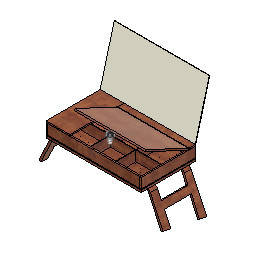
capstone new final (Autodesk Fusion 360 design; units mm, degrees)
Autodesk Fusion 360 part; units mm, degrees
note: some values were not read from the file. Set by a fixed rule: which face or edge a step refers to.
sketch "Sketch1" plane through (0, 0, 0) normal (0, 1, 0) x (1, 0, 0)
  line L0 (0, 0) -> (177.8, 0)
  line L1 (177.8, 0) -> (177.8, -406.4)
  line L2 (177.8, -406.4) -> (0, -406.4)
  line L3 (0, -406.4) -> (0, 0)
  dimension "d1" = 177.8
  dimension "d2" = 406.4
  constraint horizontal L0
  constraint vertical L1
  constraint horizontal L2
  constraint vertical L3
  constraint coincident L0.start L3.end
  measures "d1" distance of L0.start L0.end
  measures "d2" distance of L0.start L2.end
extrude "Extrude1" add sketch "Sketch1" along normal blind 12 makes body 1
extrude "Extrude2" add 1 faces at (177.8, 4, 135.4667) along direction (1, 0, 0) blind 533.4 separate body on bodies 1 makes body 2
move_face "OffsetFaces1" offset -50.8 1 faces at (355.6, 4, 0) on bodies 2
extrude "Extrude3" add 1 faces at (355.6, 4, 50.8) along direction (0, 0, -1) blind 50.8 separate body on bodies 2 makes body 3
sketch "Sketch2" plane through (0, 0, 0) normal (0, -1, 0) x (1, 0, 0)
  line L0 (177.8, 406.4) -> (0, 406.4)
  line L1 (0, 406.4) -> (0, 0)
  line L2 (0, 0) -> (177.8, 0)
  line L3 (177.8, 0) -> (177.8, 406.4)
  line L4 (0, 406.4) -> (12, 406.4)
  line L5 (12, 406.4) -> (12, 0)
  line L6 (12, 0) -> (0, 0)
  line L7 (0, 0) -> (0, 406.4)
  dimension "d10" = 12
  dimension "d11" = 406.4
  constraint horizontal L4
  constraint vertical L5
  constraint horizontal L6
  constraint vertical L7
  constraint coincident L0.end L1.start
  measures "d10" distance of L0.end L4.end
  measures "d11" distance of L0.end L1.end
extrude "Extrude4" add sketch "Sketch2" along normal blind 76.2 separate body contours L0 L1 L2 L4 L5 L6 L7 makes body 4
ref_plane "WorkPlane1" through (355.6, 6, 203.2) normal (-1, 0, 0) x (0, 0, 1)
mirror "Mirror1" about plane through (355.6, 6, 203.2) normal (-1, 0, 0) of bodies 4 makes body 5
sketch "Sketch3" plane through (0, 0, 0) normal (0, -1, 0) x (1, 0, 0)
  line L0 (711.2, 50.8) -> (177.8, 50.8)
  line L1 (177.8, 50.8) -> (177.8, 0)
  line L2 (177.8, 0) -> (711.2, 0)
  line L3 (711.2, 0) -> (711.2, 50.8)
  line L4 (0, 0) -> (36.2396, 0)
  line L5 (36.2396, 0) -> (36.2396, 369.3683)
  line L6 (36.2396, 369.3683) -> (0, 369.3683)
  line L7 (0, 369.3683) -> (0, 0)
  line L8 (20.6379, 405.3508) -> (675.3287, 405.3508)
  line L9 (675.3287, 405.3508) -> (675.3287, 393.3508)
  line L10 (675.3287, 393.3508) -> (20.6379, 393.3508)
  line L11 (20.6379, 393.3508) -> (20.6379, 405.3508)
  line L12 (11.8338, 405.3508) -> (698.3946, 405.3508)
  line L13 (698.3946, 405.3508) -> (698.3946, 393.3508)
  line L14 (698.3946, 393.3508) -> (11.8338, 393.3508)
  line L15 (11.8338, 393.3508) -> (11.8338, 405.3508)
  dimension "d16" = 12
  constraint horizontal L4
  constraint vertical L5
  constraint horizontal L6
  constraint vertical L7
  constraint coincident L4.start L7.end
  constraint horizontal L8
  constraint vertical L9
  constraint horizontal L10
  constraint vertical L11
  constraint horizontal L12
  constraint vertical L13
  constraint horizontal L14
  constraint vertical L15
  measures "d16" distance of L8 L10
extrude "Extrude5" add sketch "Sketch3" along normal blind 76.2 separate body contours L8 L9 L10 L11 L12 L14 | L11 L12 L14 L15 | L9 L12 L13 L14 makes body 6
ref_plane "WorkPlane2" through (444.5, 6, 203.2) normal (0, 0, -1) x (-1, 0, 0)
mirror "Mirror2" about plane through (444.5, 6, 203.2) normal (0, 0, -1) of bodies 6 makes body 7
sketch "Sketch4" plane through (0, 0, 0) normal (0, 1, 0) x (1, 0, 0)
ref_plane "WorkPlane3" through (355.1142, -38.1, 7.0492) normal (0, 1, 0) x (-1, 0, 0)
sketch "Sketch5" plane through (0, 0, 0) normal (0, 1, 0) x (1, 0, 0)
  line L0 (472.5788, 451.5753) -> (-238.6212, 451.5753)
  line L1 (-238.6212, 451.5753) -> (-238.6212, 45.1753)
  line L2 (-238.6212, 45.1753) -> (472.5788, 45.1753)
  line L3 (472.5788, 45.1753) -> (472.5788, 451.5753)
  dimension "d21" = 711.2
  dimension "d22" = 406.4
  constraint horizontal L0
  constraint vertical L1
  constraint horizontal L2
  constraint vertical L3
  measures "d21" distance of L0.start L0.end
  measures "d22" distance of L0.start L2.end
extrude "Extrude6" add sketch "Sketch5" along normal blind 6 separate body makes body 8
move_body "Move1" bodies 8 to x (1, 0, 0) y (0, 1, 0) z (0, 0, 1) at (0, -77.1672, 454.3724)
move_body "Move2" bodies 8 to x (1, 0, 0) y (0, 1, 0) z (0, 0, 1) at (239.8938, -5.0258, -3.112)
extrude "Extrude7" add 1 faces at (475.4059, -82.193, 270.6185) along direction (0, -1, 0) blind 18 separate body on bodies 8 makes body 9
move_body "Move3" bodies 8 9 to x (1, 0, 0) y (0, 1, 0) z (0, 0, 1) at (-1.8025, 0, 0)
sketch "Sketch6" plane through (0, -100.193, 0) normal (0, -1, 0) x (1, 0, 0)
  line L0 (710.6701, -0.3149) -> (710.6701, 406.0851)
  line L1 (710.6701, 406.0851) -> (-0.5299, 406.0851)
  line L2 (-0.5299, 406.0851) -> (-0.5299, -0.3149)
  line L3 (-0.5299, -0.3149) -> (710.6701, -0.3149)
  line L4 (-98.6513, -2.8621) -> (-403.4513, -2.8621)
  line L5 (-403.4513, -2.8621) -> (-403.4513, 47.5823)
  line L6 (-4.9831, -2.8621) -> (-55.7831, -2.8621)
  line L7 (-149.6797, 302.2068) -> (-403.6797, 302.2068)
  line L8 (-403.6797, 302.2068) -> (-403.6797, 248.7195)
  line L9 (-403.6797, 248.7195) -> (-304.5716, 248.7195)
  line L10 (-148.6459, 248.7195) -> (-140.733, 248.7195)
  line L11 (-148.6457, 48.2483) -> (-107.1833, 48.1456)
  line L12 (-253.7726, 248.4073) -> (-250.8436, 47.939)
  line L13 (-304.5716, 248.7195) -> (-304.5716, 50.2895)
  line L14 (-253.7726, 44.9279) -> (-253.7726, 248.4073)
  line L15 (-148.6459, 248.7195) -> (-253.7726, 248.4073)
  line L16 (-148.6457, 48.2483) -> (-253.7726, 44.9279)
  line L17 (-304.5716, 50.2895) -> (-403.4513, 47.5823)
  line L18 (-403.6797, 302.2068) -> (-149.6797, 302.2068)
  line L19 (-149.6797, 302.2068) -> (-140.733, 248.7195)
  line L20 (-107.1833, 48.1456) -> (-98.6513, -2.8621)
  line L21 (-304.5716, 50.2895) -> (-308.3744, 53.8896)
  line L22 (-304.5716, 248.7195) -> (-308.8143, 244.4768)
  line L23 (-253.7726, 248.4073) -> (-241.4018, 236.1097)
  line L24 (-253.7726, 44.9279) -> (-236.2729, 63.5691)
  circle A0 centre (-251.645, 246.2923) radius 3
  circle A1 centre (-306.6929, 246.5981) radius 3
  circle A2 centre (-306.7502, 52.3519) radius 3
  circle A3 centre (-251.7193, 47.1151) radius 3
  dimension "d27" = 304.8
  dimension "d29" = 50.8
  dimension "d63" = 50.8
  dimension "d64" = 203.4794
  dimension "d65" = 254
  dimension "d177" = 45
  dimension "d178" = 45
  dimension "d179" = 45
  dimension "d180" = 45
  dimension "d181" = 6
  dimension "d182" = 6
  dimension "d183" = 6
  dimension "d184" = 6
  constraint horizontal L4
  constraint vertical L5
  constraint horizontal L6
  constraint coincident L4 L6.start
  constraint horizontal L7
  constraint vertical L8
  constraint horizontal L9
  constraint collinear L9 L10
  constraint vertical L13
  constraint vertical L14
  constraint perpendicular L8 L18
  constraint collinear L19 L20
  constraint coincident L23 A0.centre
  constraint coincident L12.start A0
  constraint midpoint L22 A1.centre
  constraint coincident L9.end A1
  constraint coincident L21 A2.centre
  constraint coincident L13.end A2
  constraint coincident L24 A3.centre
  constraint coincident L14.start A3
  measures "d27" distance of L4.start L4.end
  measures "d29" distance of L6.start L6.end
  measures "d63" distance of L12.start L9.end
  measures "d64" distance of L12.start L14.start
  measures "d65" distance of L7.end L7.start
  measures "d177" angle of L17 L21
  measures "d178" angle of L16 L24
  measures "d179" angle of L15 L23
  measures "d180" angle of L13 L22
  measures "d181" diameter of A0
  measures "d182" diameter of A3
  measures "d183" diameter of A2
  measures "d184" diameter of A1
extrude "Extrude8" add sketch "Sketch6" along normal blind 18 separate body contours L4 L5 L7 L8 L9 L10 L11 L13 L14 L15 L16 L17 L18 L19 L20 A0 A1 A2 A3 makes body 10
move_body "Move4" bodies 10 to x (1, 0, 0) y (0, 1, 0) z (0, 0, 1) at (393.2413, 0, 48.0798)
move_body "Move5" bodies 10 to x (-0.422618, -0.906308, 0) y (0.906308, -0.422618, 0) z (0, 0, 1) at (101.4474, -151.9384, 0)
ref_plane "WorkPlane4" through (5.834, -93.829, 202.8851) normal (-0.707107, 0.707107, 0) x (0, 0, -1)
mirror "Mirror3" about plane through (355.6, 6, 203.2) normal (-1, 0, 0) of bodies 10 makes body 11
copy_body "CopyPasteBodies1" bodies 10 makes body 12
move_body "Move6" bodies 12 to x (1, 0, 0) y (0, 1, 0) z (0, 0, 1) at (25.4, 0, 0)
move_body "Move7" bodies 12 to x (-0.422618, 0.906308, 0) y (-0.906308, -0.422618, 0) z (0, 0, 1) at (-33.5284, -179.3234, 0)
move_body "Move8" bodies 12 to x (1, 0, 0) y (0, 1, 0) z (0, 0, 1) at (0, 10, 0)
ref_plane "WorkPlane5" through (355.0701, -91.193, 202.8851) normal (-1, 0, 0) x (0, 0, -1)
ref_plane "WorkPlane6" through (355.0701, -91.193, 202.8851) normal (1, 0, 0) x (0, 0, 1)
mirror "Mirror4" about plane through (355.0701, -91.193, 202.8851) normal (-1, 0, 0) of bodies 12 makes body 13
combine "Combine1" operation cut target body 9 tool bodies 13
combine "Combine2" operation cut target body 9 tool bodies 12
extrude "Extrude9" cut 2 faces at (534.7397, -90.3417, 332.6458) (175.4004, -90.3417, 332.6458) along direction (0, 1, 0) blind 100 on bodies 9 bodies 9
move_body "Move9" bodies 2 to x (1, 0, 0) y (0, 0.906308, -0.422618) z (0, 0.422618, 0.906308) at (0, -21.469, 4.7596)
sketch "Sketch8" plane through (0, 0, 0) normal (0, 1, 0) x (1, 0, 0)
  line L0 (-840.3694, 424.7877) -> (-129.1694, 424.7877)
  line L1 (-129.1694, 424.7877) -> (-129.1694, 18.3877)
  line L2 (-129.1694, 18.3877) -> (-840.3694, 18.3877)
  line L3 (-840.3694, 18.3877) -> (-840.3694, 424.7877)
  dimension "d46" = 711.2
  dimension "d47" = 406.4
  constraint horizontal L0
  constraint vertical L1
  constraint horizontal L2
  constraint vertical L3
  measures "d46" distance of L0.start L0.end
  measures "d47" distance of L0.start L2.end
extrude "Extrude10" add sketch "Sketch8" along normal blind 6 separate body makes body 14
move_body "Move10" bodies 14 to x (1, 0, 0) y (0, 1, 0) z (0, 0, 1) at (839.4974, 12.4407, 425.166)
move_body "Move11" bodies 14 to x (1, 0, 0) y (0, -0.258819, -0.965926) z (0, 0.965926, -0.258819) at (0, 15.2951, 12.493)
sketch "Sketch10" plane through (0, 0, 13.0492) normal (0, 0, 1) x (1, 0, 0)
  line L0 (698.3946, 0) -> (11.8338, 0)
  line L1 (11.8338, 0) -> (11.8338, -76.2)
  line L2 (11.8338, -76.2) -> (698.3946, -76.2)
  line L3 (698.3946, -76.2) -> (698.3946, 0)
  line L4 (11.8338, 0) -> (316.6338, 0)
  line L5 (316.6338, 0) -> (322.6338, 0)
  line L6 (322.6338, 0) -> (322.6338, -76.2)
  line L7 (322.6338, -76.2) -> (316.6338, -76.2)
  line L8 (316.6338, -76.2) -> (316.6338, 0)
  dimension "d51" = 304.8
  dimension "d52" = 6
  constraint coincident L0.end L1.start
  constraint perpendicular L1 L4
  constraint horizontal L5
  constraint vertical L6
  constraint horizontal L7
  constraint vertical L8
  measures "d51" distance of L0.end L4.end
  measures "d52" distance of L4.end L5.end
extrude "Extrude11" add sketch "Sketch10" along normal blind 380.238 separate body contours L0 L2 L5 L6 L7 L8 makes body 15
sketch "Sketch12" plane through (316.6338, 0, 0) normal (-1, 0, 0) x (0, 0, 1)
  line L0 (13.0492, 0) -> (13.0492, -76.2)
  line L1 (13.0492, -76.2) -> (393.2872, -76.2)
  line L2 (393.2872, -76.2) -> (393.2872, 0)
  line L3 (393.2872, 0) -> (13.0492, 0)
  line L4 (13.0492, 0) -> (241.6492, 0)
  line L5 (241.6492, 0) -> (247.6492, 0)
  line L6 (247.6492, 0) -> (247.6492, -76.2)
  line L7 (247.6492, -76.2) -> (241.6492, -76.2)
  line L8 (241.6492, -76.2) -> (241.6492, 0)
  line L9 (241.6492, 0) -> (247.6492, 0)
  line L10 (247.6492, 0) -> (247.6492, -35.3074)
  line L11 (247.6492, -35.3074) -> (241.6492, -35.3074)
  line L12 (241.6492, -35.3074) -> (241.6492, 0)
  dimension "d55" = 228.6
  dimension "d56" = 6
  constraint coincident L0.start L3.end
  constraint perpendicular L0 L4
  constraint horizontal L5
  constraint vertical L6
  constraint horizontal L7
  constraint vertical L8
  constraint horizontal L9
  constraint vertical L10
  constraint horizontal L11
  constraint vertical L12
  constraint coincident L6 L10.end
  measures "d55" distance of L0.start L4.end
  measures "d56" distance of L4.end L5.end
extrude "Extrude12" add sketch "Sketch12" along normal blind 304.6222 and the other way blind 382.524 separate body contours L3 L5 L6 L8 L9 L10 L11 L12 | L1 L6 L7 L8 L11 makes body 16
extrude "Extrude13" cut sketch "Sketch12" against normal blind 6 contours L3 L5 L6 L8 L9 L10 L11 L12 bodies 15
combine "Combine3" operation cut target body 16 tool bodies 15 keep tools
copy_body "CopyPasteBodies2" bodies 15 makes body 17
move_body "Move12" bodies 17 to x (1, 0, 0) y (0, 1, 0) z (0, 0, 1) at (190.5, 0, 0)
combine "Combine4" operation cut target body 16 tool bodies 17 keep tools
sketch "Sketch13" plane through (0, 0, 0) normal (0, 1, 0) x (1, 0, 0)
  line L0 (-304.8, -635) -> (-2743.2, -635)
  line L1 (-2743.2, -635) -> (-2743.2, 1193.8)
  line L2 (-2743.2, 1193.8) -> (-304.8, 1193.8)
  line L3 (-304.8, 1193.8) -> (-304.8, -635)
  dimension "d66" = 2438.4
  dimension "d67" = 1828.8
  constraint horizontal L0
  constraint vertical L1
  constraint horizontal L2
  constraint vertical L3
  measures "d66" distance of L0.start L0.end
  measures "d67" distance of L0.start L2.end
fillet "Fillet1" radius 31.75 4 edges at (-1.3569, -92.7345, 70.4399) (-1.2604, -92.5275, 323.543) (712.5569, -92.7345, 70.4399) (712.4604, -92.5275, 323.543) on bodies 10 11
copy_body "Body->Comp1" bodies 1 removing the originals makes body 18 in component "Component"
copy_body "Body->Comp2" bodies 3 removing the originals makes body 19 in component "Component'"
copy_body "Body->Comp3" bodies 4 removing the originals makes body 20 in component "Component''"
copy_body "Body->Comp4" bodies 5 removing the originals makes body 21 in component "Component'''"
copy_body "Body->Comp5" bodies 2 removing the originals makes body 22 in component "Component''''"
copy_body "Body->Comp6" bodies 6 removing the originals makes body 23 in component "Component'''''"
copy_body "Body->Comp7" bodies 7 removing the originals makes body 24 in component "Component''''''"
copy_body "Body->Comp8" bodies 8 removing the originals makes body 25 in component "Component'''''''"
copy_body "Body->Comp9" bodies 9 removing the originals makes body 26 in component "Component''''''''"
copy_body "Body->Comp10" bodies 10 removing the originals makes body 27 in component "Component'''''''''"
copy_body "Body->Comp12" bodies 14 removing the originals makes body 28 in component "Component''''''''''"
copy_body "Body->Comp13" bodies 15 removing the originals makes body 29 in component "Component'''''''''''"
copy_body "Body->Comp14" bodies 16 removing the originals makes body 30 in component "Component''''''''''''"
other "Arrange1"
copy_body "Body->Comp16" bodies 17 removing the originals makes body 31 in component "Component'''''''''''''"
sketch "Sketch15" plane through (0, -82.193, 0) normal (0, 1, 0) x (-1, 0, 0)
  line L0 (-520.1048, 292.2571) -> (-520.1048, 97.3822)
  line L1 (-515.8643, 93.1416) -> (-414.978, 96.3282)
  line L2 (-295.1621, 96.3282) -> (-194.2758, 93.1416)
  line L3 (-190.0353, 97.3822) -> (-190.0353, 292.2571)
  line L4 (-710.6701, 406.0851) -> (-710.6701, -0.3149)
  line L5 (-710.6701, -0.3149) -> (0.5299, -0.3149)
  line L6 (0.5299, -0.3149) -> (0.5299, 406.0851)
  line L7 (0.5299, 406.0851) -> (-710.6701, 406.0851)
  line L8 (-669.9545, 350.3046) -> (-662.1038, 342.4539)
  circle A0 centre (-667.8332, 348.1833) radius 3
  line L9 (-669.9553, 296.75) -> (-654.8973, 314.5618)
  circle A1 centre (-668.0184, 299.041) radius 3
  line L10 (-415.9545, 350.3046) -> (-437.7812, 324.5675)
  circle A2 centre (-417.8949, 348.0166) radius 3
  line L11 (-408.663, 298.3184) -> (-414.9749, 305.8746)
  circle A3 centre (-409.2513, 299.0227) radius 3
  line L12 (-669.7856, 96.0183) -> (-650.1034, 76.3361)
  line L13 (-669.7856, 45.2183) -> (-655.8865, 59.1174)
  line L14 (-364.9856, 45.2183) -> (-369.5684, 49.091)
  line L15 (-373.4724, 96.0183) -> (-388.308, 78.5248)
  line L16 (-336.6677, 96.0183) -> (-324.6859, 81.8899)
  line L17 (-345.1545, 45.2183) -> (-340.5718, 49.091)
  line L18 (-40.3545, 45.2183) -> (-57.4494, 62.3131)
  line L19 (-40.3545, 96.0183) -> (-44.5975, 91.7759)
  line L20 (-294.1856, 350.3046) -> (-290.3048, 345.7286)
  line L21 (-303.1022, 296.8276) -> (-288.6581, 311.3962)
  line L22 (-40.1856, 350.3046) -> (-44.4282, 346.0619)
  line L23 (-40.1241, 296.7773) -> (-57.2566, 316.5756)
  circle A4 centre (-667.6643, 93.897) radius 3
  circle A5 centre (-667.6643, 47.3396) radius 3
  circle A6 centre (-375.4128, 93.7303) radius 3
  circle A7 centre (-367.277, 47.1547) radius 3
  circle A8 centre (-334.7273, 93.7303) radius 3
  circle A9 centre (-342.8632, 47.1547) radius 3
  circle A10 centre (-42.476, 93.8971) radius 3
  circle A11 centre (-42.4759, 47.3396) radius 3
  circle A12 centre (-292.2452, 348.0166) radius 3
  circle A13 centre (-300.99, 298.958) radius 3
  circle A14 centre (-42.3069, 348.1833) radius 3
  circle A15 centre (-42.0872, 299.0458) radius 3
  line L24 (-520.1048, 292.2571) -> (-525.1478, 292.2571)
  line L25 (-525.1478, 292.2571) -> (-525.1478, 303.9335)
  line L26 (-525.1478, 303.9335) -> (-520.1048, 303.9335)
  line L27 (-520.1048, 303.9335) -> (-520.1048, 292.2571)
  line L28 (-520.1048, 97.3822) -> (-522.1139, 97.3822)
  line L29 (-522.1139, 97.3822) -> (-522.1139, 89.9145)
  line L30 (-522.1139, 89.9145) -> (-520.1048, 89.9145)
  line L31 (-520.1048, 89.9145) -> (-520.1048, 97.3822)
  line L32 (-521.9102, 89.8746) -> (-515.8643, 89.8746)
  line L33 (-515.8643, 89.8746) -> (-515.8643, 93.1416)
  line L34 (-515.8643, 93.1416) -> (-521.9102, 93.1416)
  line L35 (-521.9102, 93.1416) -> (-521.9102, 89.8746)
  line L36 (-187.5405, 298.6226) -> (-187.5405, 300.0194)
  line L37 (-190.0353, 292.2571) -> (-187.5405, 292.2571)
  line L38 (-187.5405, 292.2571) -> (-187.5405, 300.0194)
  line L39 (-187.5405, 300.0194) -> (-190.0353, 300.0194)
  line L40 (-190.0353, 300.0194) -> (-190.0353, 292.2571)
  line L41 (-190.0353, 97.3822) -> (-187.6059, 97.3822)
  line L42 (-187.6059, 97.3822) -> (-187.6059, 88.6357)
  line L43 (-187.6059, 88.6357) -> (-190.0353, 88.6357)
  line L44 (-190.0353, 88.6357) -> (-190.0353, 97.3822)
  line L45 (-194.2758, 93.1416) -> (-187.6059, 93.1416)
  line L46 (-187.6059, 93.1416) -> (-187.6059, 88.6357)
  line L47 (-187.6059, 88.6357) -> (-194.2758, 88.6357)
  line L48 (-194.2758, 88.6357) -> (-194.2758, 93.1416)
  arc A16 (-520.1048, 97.3822) -> (-515.8643, 93.1416) centre (-518.0515, 95.1949) ccw
  line L49 (-414.978, 96.3282) -> (-373.5155, 96.2254)
  line L50 (-373.5155, 96.2254) -> (-364.9835, 45.2177)
  line L51 (-364.9835, 45.2177) -> (-669.7835, 45.2177)
  line L52 (-669.7835, 45.2177) -> (-669.7835, 95.6622)
  line L53 (-669.7835, 95.6622) -> (-575.1449, 98.2532)
  arc A17 (-575.1449, 98.2532) -> (-570.9039, 102.4943) centre (-573.0824, 100.4318) ccw
  line L54 (-570.9039, 102.4943) -> (-570.9039, 292.5567)
  arc A18 (-570.9039, 292.5567) -> (-575.1465, 296.7993) centre (-573.0252, 294.678) ccw
  line L55 (-575.1465, 296.7993) -> (-670.012, 296.7993)
  line L56 (-670.012, 296.7993) -> (-670.012, 350.2867)
  line L57 (-670.012, 350.2867) -> (-416.012, 350.2867)
  line L58 (-416.012, 350.2867) -> (-407.0652, 296.7993)
  line L59 (-407.0652, 296.7993) -> (-414.9781, 296.7993)
  line L60 (-414.9781, 296.7993) -> (-515.8622, 296.4997)
  arc A19 (-515.8622, 296.4997) -> (-520.1048, 292.2571) centre (-517.9772, 294.3721) ccw
  arc A20 (-190.0353, 292.2571) -> (-194.2779, 296.4997) centre (-192.1629, 294.3721) ccw
  line L61 (-194.2779, 296.4997) -> (-295.162, 296.7993)
  line L62 (-295.162, 296.7993) -> (-303.0749, 296.7993)
  line L63 (-303.0749, 296.7993) -> (-294.1282, 350.2867)
  line L64 (-294.1282, 350.2867) -> (-40.1282, 350.2867)
  line L65 (-40.1282, 350.2867) -> (-40.1282, 296.7993)
  line L66 (-40.1282, 296.7993) -> (-134.9936, 296.7993)
  arc A21 (-134.9936, 296.7993) -> (-139.2363, 292.5567) centre (-137.1149, 294.678) ccw
  line L67 (-139.2363, 292.5567) -> (-139.2363, 102.4943)
  arc A22 (-139.2363, 102.4943) -> (-134.9952, 98.2532) centre (-137.0577, 100.4318) ccw
  line L68 (-134.9952, 98.2532) -> (-40.3566, 95.6622)
  line L69 (-40.3566, 95.6622) -> (-40.3566, 45.2177)
  line L70 (-40.3566, 45.2177) -> (-345.1566, 45.2177)
  line L71 (-345.1566, 45.2177) -> (-336.6246, 96.2254)
  line L72 (-336.6246, 96.2254) -> (-295.1621, 96.3282)
  arc A23 (-194.2758, 93.1416) -> (-190.0353, 97.3822) centre (-192.0886, 95.1949) ccw
  line L73 (-194.2779, 296.4997) -> (-187.5405, 296.4997)
  line L74 (-187.5405, 296.4997) -> (-187.5405, 300.0194)
  line L75 (-187.5405, 300.0194) -> (-194.2779, 300.0194)
  line L76 (-194.2779, 300.0194) -> (-194.2779, 296.4997)
  line L77 (-139.2363, 292.5567) -> (-141.4028, 292.5567)
  line L78 (-141.4028, 292.5567) -> (-141.4028, 299.9763)
  line L79 (-141.4028, 299.9763) -> (-139.2363, 299.9763)
  line L80 (-139.2363, 299.9763) -> (-139.2363, 292.5567)
  line L81 (-134.9936, 296.7993) -> (-141.4028, 296.7993)
  line L82 (-141.4028, 296.7993) -> (-141.4028, 299.9763)
  line L83 (-141.4028, 299.9763) -> (-134.9936, 299.9763)
  line L84 (-134.9936, 299.9763) -> (-134.9936, 296.7993)
  line L85 (-134.9952, 98.2532) -> (-142.1795, 98.2532)
  line L86 (-142.1795, 98.2532) -> (-142.1795, 95.2836)
  line L87 (-142.1795, 95.2836) -> (-134.9952, 95.2836)
  line L88 (-134.9952, 95.2836) -> (-134.9952, 98.2532)
  line L89 (-139.2363, 102.4943) -> (-142.1795, 102.4943)
  line L90 (-142.1795, 102.4943) -> (-142.1795, 95.2836)
  line L91 (-142.1795, 95.2836) -> (-139.2363, 95.2836)
  line L92 (-139.2363, 95.2836) -> (-139.2363, 102.4943)
  line L93 (-570.9039, 102.4943) -> (-568.96, 102.4943)
  line L94 (-568.96, 102.4943) -> (-568.96, 93.98)
  line L95 (-568.96, 93.98) -> (-570.9039, 93.98)
  line L96 (-570.9039, 93.98) -> (-570.9039, 102.4943)
  line L97 (-575.1449, 98.2532) -> (-568.96, 98.2532)
  line L98 (-568.96, 98.2532) -> (-568.96, 93.98)
  line L99 (-568.96, 93.98) -> (-575.1449, 93.98)
  line L100 (-575.1449, 93.98) -> (-575.1449, 98.2532)
  line L101 (-515.8622, 296.4997) -> (-525.1478, 296.4997)
  line L102 (-525.1478, 296.4997) -> (-525.1478, 303.9335)
  line L103 (-525.1478, 303.9335) -> (-515.8622, 303.9335)
  line L104 (-515.8622, 303.9335) -> (-515.8622, 296.4997)
  line L105 (-570.9039, 292.5567) -> (-568.96, 292.5567)
  line L106 (-568.96, 292.5567) -> (-568.96, 299.72)
  line L107 (-568.96, 299.72) -> (-570.9039, 299.72)
  line L108 (-570.9039, 299.72) -> (-570.9039, 292.5567)
  line L109 (-575.1465, 296.7993) -> (-568.96, 296.7993)
  line L110 (-568.96, 296.7993) -> (-568.96, 299.72)
  line L111 (-568.96, 299.72) -> (-575.1465, 299.72)
  line L112 (-575.1465, 299.72) -> (-575.1465, 296.7993)
  dimension "d144" = 6
  dimension "d146" = 6
  dimension "d148" = 6
  dimension "d150" = 6
  dimension "d163" = 6
  dimension "d164" = 6
  dimension "d165" = 6
  dimension "d166" = 6
  dimension "d167" = 6
  dimension "d168" = 6
  dimension "d169" = 6
  dimension "d170" = 6
  dimension "d171" = 6
  dimension "d172" = 6
  dimension "d173" = 6
  dimension "d174" = 6
  constraint coincident L8 A0.centre
  constraint coincident L8.start A0
  constraint coincident L9 A1.centre
  constraint coincident L9.start A1
  constraint coincident L10 A2.centre
  constraint coincident L11 A3.centre
  constraint coincident L12 A4.centre
  constraint coincident L12.start A4
  constraint coincident L13 A5.centre
  constraint coincident L15 A6.centre
  constraint coincident L15.start A6
  constraint midpoint L14 A7.centre
  constraint coincident L14.start A7
  constraint coincident L16 A8.centre
  constraint coincident L16.start A8
  constraint midpoint L17 A9.centre
  constraint coincident L17.start A9
  constraint midpoint L19 A10.centre
  constraint coincident L19.start A10
  constraint coincident L18 A11.centre
  constraint coincident L18.start A11
  constraint midpoint L20 A12.centre
  constraint coincident L20.start A12
  constraint coincident L21 A13.centre
  constraint coincident L21.start A13
  constraint midpoint L22 A14.centre
  constraint coincident L22.start A14
  constraint coincident L23 A15.centre
  constraint coincident L23.start A15
  constraint horizontal L24
  constraint vertical L25
  constraint horizontal L26
  constraint vertical L27
  constraint coincident L0.start L24.start
  constraint horizontal L28
  constraint vertical L29
  constraint horizontal L30
  constraint vertical L31
  constraint coincident L0.end L28.start
  constraint horizontal L32
  constraint vertical L33
  constraint horizontal L34
  constraint vertical L35
  constraint coincident L1.start L33.end
  constraint vertical L36
  constraint horizontal L37
  constraint vertical L38
  constraint horizontal L39
  constraint vertical L40
  constraint coincident L3.end L37.start
  constraint horizontal L41
  constraint vertical L42
  constraint horizontal L43
  constraint vertical L44
  constraint coincident L3.start L41.start
  constraint horizontal L45
  constraint vertical L46
  constraint horizontal L47
  constraint vertical L48
  constraint coincident L2.end L45.start
  constraint horizontal L73
  constraint vertical L74
  constraint horizontal L75
  constraint vertical L76
  constraint coincident A20.end L61.start
  constraint horizontal L77
  constraint vertical L78
  constraint horizontal L79
  constraint vertical L80
  constraint coincident A21.end L67.start
  constraint horizontal L81
  constraint vertical L82
  constraint horizontal L83
  constraint vertical L84
  constraint coincident L66.end A21.start
  constraint horizontal L85
  constraint vertical L86
  constraint horizontal L87
  constraint vertical L88
  constraint coincident A22.end L68.start
  constraint horizontal L89
  constraint vertical L90
  constraint horizontal L91
  constraint vertical L92
  constraint coincident L67.end A22.start
  constraint horizontal L93
  constraint vertical L94
  constraint horizontal L95
  constraint vertical L96
  constraint coincident A17.end L54.start
  constraint horizontal L97
  constraint vertical L98
  constraint horizontal L99
  constraint vertical L100
  constraint coincident L53.end A17.start
  constraint horizontal L101
  constraint vertical L102
  constraint horizontal L103
  constraint vertical L104
  constraint coincident L60.end A19.start
  constraint horizontal L105
  constraint vertical L106
  constraint horizontal L107
  constraint vertical L108
  constraint coincident L54.end A18.start
  constraint horizontal L109
  constraint vertical L110
  constraint horizontal L111
  constraint vertical L112
  constraint coincident A18.end L55.start
  measures "d144" diameter of A0
  measures "d146" diameter of A1
  measures "d148" diameter of A2
  measures "d150" diameter of A3
  measures "d163" diameter of A4
  measures "d164" diameter of A5
  measures "d165" diameter of A6
  measures "d166" diameter of A7
  measures "d167" diameter of A8
  measures "d168" diameter of A9
  measures "d169" diameter of A10
  measures "d170" diameter of A11
  measures "d171" diameter of A12
  measures "d172" diameter of A13
  measures "d173" diameter of A14
  measures "d174" diameter of A15
extrude "Extrude2'" cut sketch "Sketch15" against normal blind 25.4 contours L27 A19 | L24 L25 L27 A19 L101 | L28 L29 L30 L34 L35 A16 | L31 L34 A16 | L27 A19 L101 | L31 L34 A16 | L31 L34 A16 | L30 L31 L34 L35 A16 | L25 L26 L27 L101 L102 L103 | L27 A19 L101 L103 L104 | A19 L101 | L30 L31 L32 L33 L35 A16 | L15 A6 L49 L50 | A6 L49 | A3 L59 | A3 L58 L59 | L15 A6 L50 | L15 A6 L50 | L15 A6 L50 | A3 L58 | L14 A7 L50 | A7 L50 | L10 A2 L58 | L10 A2 L58 | L14 A7 L51 | A7 L51 | L10 A2 L57 L58 | L10 A2 L57 L58 | L13 A5 L51 | A5 L51 | L8 A0 L57 | L8 A0 L57 | L13 A5 L52 | A5 L52 | L8 A0 L57 | L8 A0 L56 L57 | L12 A4 L52 L53 | L12 A4 L52 L53 | A0 L56 | L12 A4 L53 | L12 A4 L53 | A1 L56 | L9 A1 L55 L56 | L9 A1 L55 | L9 A1 L55 | A17 L97 | A17 L96 L97 L99 L100 | L9 A1 L55 | A17 L96 | A17 L93 L94 L96 L97 | L94 L95 L96 L97 L98 L99 | A18 L108 L111 L112 | A18 L109 | A18 L105 L106 L109 | A18 L108 | L106 L107 L108 L109 L110 L111 | L44 L47 L48 A23 | L44 L45 A23 | A8 L72 | L16 A8 L71 L72 | L44 L45 A23 | L44 L45 A23 | L42 L43 L44 L45 L46 L47 A23 | L41 L42 L45 A23 | L16 A8 L71 | L16 A8 L71 | L37 L38 L40 A20 L73 | L40 A20 | L16 A8 L71 | L40 A20 L73 | A9 L71 | L17 A9 L71 | L36 L38 L39 L40 L73 L74 L75 | L40 A20 L73 L75 L76 | A20 L73 | L17 A9 L70 | A9 L70 | A11 L70 | L18 A11 L70 | L21 A13 L62 L63 | A13 L62 | L18 A11 L69 | A11 L69 | L21 A13 L63 | L21 A13 L63 | L21 A13 L63 | L19 A10 L68 L69 | L19 A10 L68 L69 | L19 A10 L68 | L20 A12 L63 | L20 A12 L63 | L19 A10 L68 | L20 A12 L63 L64 | L20 A12 L63 L64 | A22 L85 L87 L88 L92 | A22 L85 | L22 A14 L64 | L22 A14 L64 | A22 L85 L89 L90 L92 | A22 L92 | L85 L86 L87 L90 L91 L92 | L22 A14 L64 | L22 A14 L64 L65 | A14 L65 | A21 L77 L78 L81 | A21 L80 | L23 A15 L65 L66 | L23 A15 L65 L66 | A21 L80 L83 L84 | L78 L79 L80 L81 L82 L83 | A21 L81 | L23 A15 L66 | L23 A15 L66 picked at (-409.0286, 299.5198) bodies 26 in component "Component''''''''"
copy_body "Body->Comp17" bodies 11 removing the originals makes body 32 in component "Component''''''''''''''"
other "Arrange3"
sketch "Sketch16" plane through (316.6338, 0, 0) normal (-1, 0, 0) x (0, 0, 1)
  line L0 (241.6492, -35.3074) -> (241.6492, 0)
  line L1 (241.6492, 0) -> (13.0492, 0)
  line L2 (13.0492, 0) -> (13.0492, -76.2)
  line L3 (13.0492, -76.2) -> (393.2872, -76.2)
  line L4 (393.2872, -76.2) -> (393.2872, 0)
  line L5 (393.2872, 0) -> (247.6492, 0)
  line L6 (247.6492, 0) -> (247.6492, -35.3074)
  line L7 (247.6492, -35.3074) -> (241.6492, -35.3074)
  circle A0 centre (244.6492, -35.3074) radius 3
  line L8 (241.6492, 0) -> (247.8492, 0)
  line L9 (247.8492, 0) -> (247.8492, -35.3074)
  line L10 (247.8492, -35.3074) -> (241.6492, -35.3074)
  line L11 (241.6492, -35.3074) -> (241.6492, 0)
  dimension "d250" = 6.2
  constraint tangent L0 A0
  constraint horizontal L8
  constraint vertical L9
  constraint horizontal L10
  constraint vertical L11
  constraint coincident L0.end L1.start
  measures "d250" distance of L0.end L8.end
sketch "Sketch17" plane through (0, 0, 247.6492) normal (0, 0, 1) x (1, 0, 0)
  line L0 (699.1578, 0) -> (12.0116, 0)
  line L1 (12.0116, 0) -> (12.0116, -76.2)
  line L2 (12.0116, -76.2) -> (316.6338, -76.2)
  line L3 (316.6338, -76.2) -> (316.6338, -35.3074)
  line L4 (316.6338, -35.3074) -> (322.6338, -35.3074)
  line L5 (322.6338, -35.3074) -> (322.6338, -76.2)
  line L6 (322.6338, -76.2) -> (507.1338, -76.2)
  line L7 (507.1338, -76.2) -> (507.1338, -35.3074)
  line L8 (507.1338, -35.3074) -> (513.1338, -35.3074)
  line L9 (513.1338, -35.3074) -> (513.1338, -76.2)
  line L10 (513.1338, -76.2) -> (699.1578, -76.2)
  line L11 (699.1578, -76.2) -> (699.1578, 0)
  circle A0 centre (319.6338, -35.2018) radius 3.0019
  circle A1 centre (510.1338, -35.3074) radius 3
  line L12 (316.6338, -76.2) -> (322.7338, -76.2)
  line L13 (322.7338, -76.2) -> (322.7338, -35.3074)
  line L14 (322.7338, -35.3074) -> (316.6338, -35.3074)
  line L15 (316.6338, -35.3074) -> (316.6338, -76.2)
  line L16 (507.1338, -76.2) -> (513.3338, -76.2)
  line L17 (513.3338, -76.2) -> (513.3338, -35.3074)
  line L18 (513.3338, -35.3074) -> (507.1338, -35.3074)
  line L19 (507.1338, -35.3074) -> (507.1338, -76.2)
  dimension "d248" = 6.1
  dimension "d249" = 6.2
  constraint coincident L4.end A0
  constraint coincident L7.end A1
  constraint tangent L7 A1
  constraint coincident L8.end A1
  constraint horizontal L12
  constraint vertical L13
  constraint horizontal L14
  constraint vertical L15
  constraint coincident L2.end L3.start
  constraint horizontal L16
  constraint vertical L17
  constraint horizontal L18
  constraint vertical L19
  constraint coincident L6.end L7.start
  measures "d248" distance of L2.end L12.end
  measures "d249" distance of L6.end L16.end
extrude "Extrude1'" cut sketch "Sketch17" against normal blind 7.62 contours L9 L10 L16 L17 L18 | L3 L5 A0 L12 L15 | L7 L9 A1 L16 L19 | L4 A0 L14 | L4 A0 L14 | L5 L6 L12 L13 L14 | L8 A1 L18 | L8 A1 L18 bodies 30 in component "Component''''''''''''"
extrude "Extrude2''" cut sketch "Sketch16" against normal blind 203.2 contours L7 A0 L10 | L0 L6 A0 L8 L11 | L7 A0 L10 | L5 L6 L8 L9 L10 bodies 29 in component "Component'''''''''''"
extrude "Extrude2'''" cut sketch "Sketch16" against normal blind 203.2 contours L7 A0 L10 | L0 L6 A0 L8 L11 | L7 A0 L10 | L5 L6 L8 L9 L10 bodies 31 in component "Component'''''''''''''"
other "Arrange4"
sketch "Sketch19" plane through (0, 0, 0) normal (0, 1, 0) x (1, 0, 0)
  line L0 (-3000.7449, 1512.9384) -> (3967.3165, 1512.9384)
  line L1 (3967.3165, 1512.9384) -> (3967.3165, -1853.7265)
  line L2 (3967.3165, -1853.7265) -> (-3000.7449, -1853.7265)
  line L3 (-3000.7449, -1853.7265) -> (-3000.7449, 1512.9384)
  constraint horizontal L0
  constraint vertical L1
  constraint horizontal L2
  constraint vertical L3
extrude "Extrude1''" cut sketch "Sketch19" along normal blind 2 bodies 18 in component "Component"
extrude "Extrude1'''" cut sketch "Sketch19" along normal blind 2 bodies 19 in component "Component'"
extrude "Extrude1''''" cut sketch "Sketch19" along normal blind 2 bodies 22 in component "Component''''"
extrude "Extrude1'''''" cut sketch "Sketch19" along normal blind 2 sketch seen with x (0, 0, -1) y (1, 0, 0) z (0, -1, 0) at (699.2, 202.15, 1504.95) bodies 21 in component "Component'''"
extrude "Extrude3'" cut sketch "Sketch19" along normal blind 2 sketch seen with x (0, 0, -1) y (0, 1, 0) z (1, 0, 0) at (-1022.8799, -100.193, 412.4351) bodies 26 in component "Component''''''''"
extrude "Extrude1''''''" cut sketch "Sketch19" along normal blind 2 sketch seen with x (-0.422618, -0.906308, 0) y (-0.906308, 0.422618, 0) z (0, 0, -1) at (197.0327, 290.1218, 1372.6367) bodies 27 in component "Component'''''''''"
extrude "Extrude1'''''''" cut sketch "Sketch19" along normal blind 2 sketch seen with x (0.422618, -0.906308, 0) y (0.906308, 0.422618, 0) z (0, 0, 1) at (514.1597, 290.1381, -1300.2099) bodies 32 in component "Component''''''''''''''"
extrude "Extrude1''''''''" cut sketch "Sketch19" along normal blind 2 sketch seen with x (0, 0, 1) y (0, 1, 0) z (-1, 0, 0) at (717.0201, -82.193, 1161.7351) bodies 25 in component "Component'''''''"
extrude "Extrude1'''''''''" cut sketch "Sketch19" along normal blind 2 sketch seen with x (0, 0.965926, -0.258819) y (0, 0.258819, 0.965926) z (1, 0, 0) at (-7.2221, 723.3947, -196.3329) bodies 28 in component "Component''''''''''"
extrude "Extrude3''" cut sketch "Sketch19" along normal blind 2 sketch seen with x (0, 1, 0) y (1, 0, 0) z (0, 0, -1) at (316.6338, 48.6156, 824.0458) bodies 29 in component "Component'''''''''''"
extrude "Extrude2''''" cut sketch "Sketch19" along normal blind 2 sketch seen with x (0, -1, 0) y (0, 0, 1) z (-1, 0, 0) at (705.5078, -313.2329, 241.6492) bodies 30 in component "Component''''''''''''"
extrude "Extrude3'''" cut sketch "Sketch19" along normal blind 2 sketch seen with x (0, 1, 0) y (1, 0, 0) z (0, 0, -1) at (507.1338, 142.8242, 824.0458) bodies 31 in component "Component'''''''''''''"
component "Component" placed x (1, 0, 0) y (0, 1, 0) z (0, 0, 1) at (0, 0, 0)
component "Component'" placed x (1, 0, 0) y (0, 1, 0) z (0, 0, 1) at (0, 0, 0)
component "Component''" placed x (1, 0, 0) y (0, 1, 0) z (0, 0, 1) at (0, 0, 0)
component "Component'''" placed x (1, 0, 0) y (0, 1, 0) z (0, 0, 1) at (0, 0, 0)
component "Component''''" placed x (1, 0, 0) y (0, 1, 0) z (0, 0, 1) at (0, 0, 0)
component "Component'''''" placed x (1, 0, 0) y (0, 1, 0) z (0, 0, 1) at (0, 0, 0)
component "Component''''''" placed x (1, 0, 0) y (0, 1, 0) z (0, 0, 1) at (0, 0, 0)
component "Component'''''''" placed x (1, 0, 0) y (0, 1, 0) z (0, 0, 1) at (0, 0, 0)
component "Component''''''''" placed x (1, 0, 0) y (0, 1, 0) z (0, 0, 1) at (0, 0, 0)
component "Component'''''''''" placed x (1, 0, 0) y (0, 1, 0) z (0, 0, 1) at (0, 0, 0)
component "Component''''''''''" placed x (1, 0, 0) y (0, 1, 0) z (0, 0, 1) at (0, 0, 0)
component "Component'''''''''''" placed x (1, 0, 0) y (0, 1, 0) z (0, 0, 1) at (0, 0, 0)
component "Component''''''''''''" placed x (1, 0, 0) y (0, 1, 0) z (0, 0, 1) at (0, 0, 0)
component "Arrange1" placed x (1, 0, 0) y (0, 1, 0) z (0, 0, 1) at (0, 0, 0)
component "Component'''''''''''''" placed x (1, 0, 0) y (0, 1, 0) z (0, 0, 1) at (0, 0, 0)
component "Component''''''''''''''" placed x (1, 0, 0) y (0, 1, 0) z (0, 0, 1) at (0, 0, 0)
component "Arrange3" placed x (1, 0, 0) y (0, 1, 0) z (0, 0, 1) at (0, 0, 0)
component "Arrange4" placed x (1, 0, 0) y (0, 1, 0) z (0, 0, 1) at (0, 0, 0)
component "Envelope1(Qty: 1)" placed x (0, 0, 1) y (1, 0, 0) z (0, 1, 0) at (1092.2, 0, 0) in component "Arrange1"
component "Component" placed x (1, 0, 0) y (0, 0, 1) z (0, -1, 0) at (6.35, 412.75, 0) in component "Envelope1(Qty: 1)"
component "Component'''" placed x (0, 0, 1) y (-1, 0, 0) z (0, -1, 0) at (202.15, 412.75, -699.2) in component "Envelope1(Qty: 1)"
component "Envelope1(Qty: 1) (1)" placed x (0, 0, 1) y (1, 0, 0) z (0, 1, 0) at (0, 0, 1016) in component "Arrange3"
component "Component''''''''" placed x (1, 0, 0) y (0, 0, 1) z (0, -1, 0) at (6.8799, 412.4351, 100.193) in component "Envelope1(Qty: 1) (1)"
component "Component'''''''''" placed x (0, -0.422618, -0.906308) y (0, -0.906308, 0.422618) z (-1, 0, 0) at (356.6367, 346.2092, 55.9615) in component "Envelope1(Qty: 1) (1)"
component "Component''''''''''''''" placed x (0, 0.422618, 0.906308) y (0, -0.906308, 0.422618) z (1, 0, 0) at (284.2099, 45.6612, -588.6046) in component "Envelope1(Qty: 1) (1)"
component "Envelope1(Qty: 1) (2)" placed x (0, 0, 1) y (1, 0, 0) z (0, 1, 0) at (-1168.4, 0, 0) in component "Arrange4"
component "Component'''''''" placed x (-1, 0, 0) y (0, 0, 1) z (0, 1, 0) at (717.0201, 6.6649, 82.193) in component "Envelope1(Qty: 1) (2)"
component "Component''''''''''" placed x (1, 0, 0) y (0, 0.965926, 0.258819) z (0, -0.258819, 0.965926) at (7.2221, 418.8397, 2.4147) in component "Envelope1(Qty: 1) (2)"
component "Component''''''''''''" placed x (-1, 0, 0) y (0, -1, 0) z (0, 0, 1) at (705.5078, 855.1671, -241.6492) in component "Envelope1(Qty: 1) (2)"
component "Component" placed x (0, 1, 0) y (0, 0, 1) z (1, 0, 0) at (6.35, 949.3757, 0) in component "Envelope1(Qty: 1) (2)"
component "Component'''''''''''" placed x (0, 0, 1) y (0, 1, 0) z (-1, 0, 0) at (824.0458, 1119.7844, -316.6338) in component "Envelope1(Qty: 1) (2)"
component "Component'''''''''''''" placed x (0, 0, 1) y (0, 1, 0) z (-1, 0, 0) at (824.0458, 1025.5758, -507.1338) in component "Envelope1(Qty: 1) (2)"
